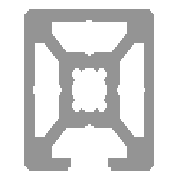
# Autodesk Inventor part: 3 842 993 421-25mm
Saved by Autodesk Inventor 2011 SP1 (Build 150282100, 282)
## iProperties
Created: 2011-02-10
Part Number: 3 842 993 421-25mm
Document SubType Name: Modeling
Designer: S. Wile
Density: 2.71 g/cm^3
Categories: <MemberInstance><Categories><Category DisplayName="Structural Shapes" InternalName="089c4875-fa83-4c05-b084-43b9cc11f5ed" Mnemonic="GRDR"><CategoryParameter DisplayName="Custom Base Point" InternalName="4f1d1b73-316d-484b-a3df-9cbabb16eb77" Mnemonic="shpBasePoint"/><CategoryParameter DisplayName="FG Authored" InternalName="9c666724-f362-4ea7-ac62-f6a007de5c69" Mnemonic="shpFGAuto"/><CategoryParameter DisplayName="Legacy Member ID" InternalName="340afe4f-75d7-48d3-ab7d-943f3c3da468" Mnemonic="LegacyMemberID"/><CategoryParameter DisplayName="Base Length" InternalName="42e34263-8f20-4d0e-ad48-bf1385b87c24" Mnemonic="shplen"/><CategoryParameter DisplayName="Distance of the Center of Gravity X-X" InternalName="26c9bdb8-9c79-4b4f-a92e-8e197583c9c4" Mnemonic="grcendistX"/><CategoryParameter DisplayName="Distance of the Center of Gravity Y-Y" InternalName="bcc4fb17-7af4-436a-8f8c-d0aa3b0248c5" Mnemonic="grcendistY"/><CategoryParameter DisplayName="Torsional Rigidity Modulus" InternalName="26c1ec35-5026-4c63-ad0a-751cf684a536" Mnemonic="torrigmod"/><CategoryParameter DisplayName="Torsional Section Modulus" InternalName="7c55a8dc-8844-49f9-a867-cc677b30ec9a" Mnemonic="torsecmod"/><CategoryParameter DisplayName="Coefficient of Shear Displacement" InternalName="de4c90c6-aaa8-468f-a335-6737b311b5d3" Mnemonic="shdispc"/><CategoryParameter DisplayName="Section Area" InternalName="1ff91680-64b0-4202-b9a3-7fd3f94bba3b" Mnemonic="secarea"/><CategoryParameter DisplayName="Moment of Inertia (x)" InternalName="4cd780bc-73d7-43ac-917a-579e5cbd684d" Mnemonic="inermomx"/><CategoryParameter DisplayName="Moment of Inertia (y)" InternalName="4b9f58ea-bced-460e-81ea-3d29ca5a49e3" Mnemonic="inermomy"/><CategoryParameter DisplayName="Section Module (x)" InternalName="72cfad18-cf51-4ed4-aaa7-c6b224f8419f" Mnemonic="secmodx"/><CategoryParameter DisplayName="Section Module (y)" InternalName="59eaa5e9-d227-48dc-b6c1-6920f96e0f95" Mnemonic="secmody"/><CategoryParameter DisplayName="Radius of Gyration (x)" InternalName="25778675-03e9-40c1-b6a8-4a9ed693320d" Mnemonic="gyrradx"/><CategoryParameter DisplayName="Radius of Gyration (y)" InternalName="bfa18ebe-1636-4dbe-8d42-b263e0b73184" Mnemonic="gyrrady"/><CategoryParameter DisplayName="Shape Thickness" InternalName="d109cf76-8eb4-42fc-9800-4409734adc67" Mnemonic="shpthick"/><CategoryParameter DisplayName="Second Shape Thickness" InternalName="9251a8e1-85fd-4e47-af99-afdb762317d9" Mnemonic="shpthick2"/><CategoryParameter DisplayName="Shape Width" InternalName="7c717d54-a18f-4666-b4d4-573cce22c62c" Mnemonic="shpwdth"/><CategoryParameter DisplayName="Shape Height" InternalName="50274e7d-5ac0-4796-92cb-c59e54983c67" Mnemonic="shpheig"/><CategoryParameter DisplayName="Mass per Length Unit" InternalName="0bb95a10-148f-4027-a459-38d7b056702a" Mnemonic="shpmass"/><CategoryParameter DisplayName="Section Designation" InternalName="5a64d034-428d-49c8-ba32-7619764de20f" Mnemonic="shpdes"/><Category DisplayName="Other" InternalName="f02205ff-2390-476f-921c-0b3185f88e84" Mnemonic="OTHSHP"><CategoryParameter DisplayName="Moment of Inertia (x)" InternalName="ec6737bc-264f-43ed-b0bd-f6d410c2718d" Mnemonic="inermomx"/><CategoryParameter DisplayName="Moment of Inertia (y)" InternalName="044c654e-f649-48ac-84cc-650a29ae31ca" Mnemonic="inermomy"/><CategoryParameter DisplayName="Section Module (x)" InternalName="cac70804-9d39-43bb-be17-56ea1f39a6c2" Mnemonic="secmodx"/><CategoryParameter DisplayName="Section Module (y)" InternalName="88b8bff9-a616-4028-93d5-ed4f79680d13" Mnemonic="secmody"/><CategoryParameter DisplayName="Section Area" InternalName="c46ecdf8-b6eb-4db9-8b25-30258930c1e3" Mnemonic="secarea"/><CategoryParameter DisplayName="Radius of Gyration (x)" InternalName="ee72c61e-565e-4fd6-b448-66e1e1abcb7e" Mnemonic="gyrradx"/><CategoryParameter DisplayName="Radius of Gyration (y)" InternalName="743e1dfe-1bba-408b-b985-cf752b207386" Mnemonic="gyrrady"/><CategoryParameter DisplayName="Shape Thickness" InternalName="12b1a788-9233-48fd-a933-2df8ff42b15f" Mnemonic="shpthick"/><CategoryParameter DisplayName="Mass per Length Unit" InternalName="2fd289d6-9394-4d2d-97e6-6659d7d4551d" Mnemonic="shpmass"/></Category></Category></Categories><FamilyTemplate Id="20x20-1S"><FamilyTemplateParameters><FamilyTemplateParameter ObjectType="kUserParameterObject" ValueType="xs:double" Id="1" ObjectReferenceKey="Length"/><FamilyTemplateParameter ObjectType="kPropertyObject" ValueType="xs:string" Id="4" ObjectReferenceKey="{32853F0F-3444-11d1-9E93-0060B03C1CA6}" SubObjectId="52"/><FamilyTemplateParameter ObjectType="kPartComponentDefinitionObject" ValueType="xs:string" Id="5" SubObjectId="Material"/><FamilyTemplateParameter ObjectType="kPropertyObject" ValueType="xs:string" Id="6" ObjectReferenceKey="{32853F0F-3444-11d1-9E93-0060B03C1CA6}" SubObjectId="5"/><FamilyTemplateParameter ObjectType="kPropertyObject" ValueType="xs:string" Id="7" ObjectReferenceKey="{32853F0F-3444-11D1-9E93-0060B03C1CA6}" SubObjectId="55"/><FamilyTemplateParameter ObjectType="kiPartTableColumnObject" ValueType="xs:string" Id="16" ObjectReferenceKey="FILENAME"/><FamilyTemplateParameter ObjectType="kiPartTableColumnObject" ValueType="xs:string" Id="17" ObjectReferenceKey="MEMBER_REVISION"/></FamilyTemplateParameters></FamilyTemplate><CategoryParameterMap><ParamToTemplateMap><ParamToTemplate CategoryParameter="//CategoryParameter[@InternalName='2675968c-4ce5-49e0-a4f5-552d29089031']" TemplateParameter="4"/><ParamToTemplate CategoryParameter="//CategoryParameter[@InternalName='8b46a4cc-9585-4fed-90c3-899f57e09a73']" TemplateParameter="16"/><ParamToTemplate CategoryParameter="//CategoryParameter[@InternalName='42e34263-8f20-4d0e-ad48-bf1385b87c24']" TemplateParameter="1"/><ParamToTemplate CategoryParameter="//CategoryParameter[@InternalName='818a152a-d3c3-49ca-80ee-df7d91421b8e']" TemplateParameter="5"/><ParamToTemplate CategoryParameter="//CategoryParameter[@InternalName='a65d44b9-392f-4f4f-857b-e4b3d54996fe']" TemplateParameter="17"/><ParamToTemplate CategoryParameter="//CategoryParameter[@InternalName='016b6077-bfbe-49bd-92c9-d8d59c39c941']" TemplateParameter="6"/><ParamToTemplate CategoryParameter="//CategoryParameter[@InternalName='9c666724-f362-4ea7-ac62-f6a007de5c69']" ConstantValue="1"/></ParamToTemplateMap></CategoryParameterMap></MemberInstance>
Stock Number: 3 842 993 421
Description: PROFILE 20x20 1S, -/-
Material: Aluminum-6061
Mass: 13.0174 g
Surface Area: 55.674 cm^2
Volume: 4.80347 cm^3
Author: S. Wile
Autodesk Inventor part; units mm, degrees
ref_plane "YZ Plane" through (0, 0, 0) normal (1, 0, 0) x (0, 1, 0)
ref_plane "XZ Plane" through (0, 0, 0) normal (0, 1, 0) x (-1, 0, 0)
ref_plane "XY Plane" through (0, 0, 0) normal (0, 0, 1) x (1, 0, 0)
sketch "20x20-1S" plane through (0, 0, 0) normal (0, 0, 1) x (1, 0, 0)
  arc A0 (162.0009, 79.9596) -> (163.0616, 81.0203) centre (160.1138, 82.9073) ccw
  line L0 (163.0616, 81.0203) -> (162.5495, 81.6306)
  arc A1 (162.5495, 81.6306) -> (162.5495, 84.184) centre (160.1138, 82.9073) ccw
  line L1 (162.5495, 84.184) -> (163.0616, 84.7943)
  arc A2 (163.0616, 84.7943) -> (162.0009, 85.855) centre (160.1138, 82.9073) ccw
  line L2 (162.0009, 85.855) -> (161.3907, 85.3429)
  arc A3 (161.3907, 85.3429) -> (158.8369, 85.3429) centre (160.1138, 82.9073) ccw
  line L3 (158.8369, 85.3429) -> (158.2267, 85.855)
  arc A4 (158.2267, 85.855) -> (157.166, 84.7943) centre (160.1138, 82.9073) ccw
  line L4 (157.166, 84.7943) -> (157.6781, 84.184)
  arc A5 (157.6781, 84.184) -> (157.6781, 81.6306) centre (160.1138, 82.9073) ccw
  line L5 (157.6781, 81.6306) -> (157.166, 81.0203)
  arc A6 (157.166, 81.0203) -> (158.2267, 79.9596) centre (160.1138, 82.9073) ccw
  line L6 (158.2267, 79.9596) -> (158.8369, 80.4717)
  arc A7 (158.8369, 80.4717) -> (161.3907, 80.4717) centre (160.1138, 82.9073) ccw
  line L7 (161.3907, 80.4717) -> (162.0009, 79.9596)
  line L8 (164.6138, 81.9877) -> (164.6138, 79.5508)
  line L9 (164.6724, 79.4094) -> (167.1159, 76.9659)
  line L10 (167.2573, 76.9073) -> (168.4138, 76.9073)
  line L11 (168.6138, 77.1073) -> (168.6138, 82.3341)
  line L12 (168.6406, 82.4341) -> (168.8561, 82.8073)
  line L13 (168.8561, 83.0073) -> (168.6406, 83.3805)
  line L14 (168.6138, 83.4805) -> (168.6138, 88.7073)
  line L15 (168.4138, 88.9073) -> (167.2573, 88.9073)
  line L16 (167.1159, 88.8487) -> (164.6724, 86.4052)
  line L17 (164.6138, 86.2638) -> (164.6138, 83.8269)
  line L18 (164.587, 83.7269) -> (164.1715, 83.0073)
  line L19 (164.1715, 82.8073) -> (164.587, 82.0877)
  line L20 (161.0334, 87.4073) -> (163.4703, 87.4073)
  line L21 (166.1138, 90.0508) -> (166.1138, 91.2073)
  line L22 (165.9138, 91.4073) -> (160.687, 91.4073)
  line L23 (160.587, 91.4341) -> (160.2138, 91.6495)
  line L24 (160.0138, 91.6495) -> (159.6406, 91.4341)
  line L25 (159.5406, 91.4073) -> (154.3138, 91.4073)
  line L26 (154.1138, 91.2073) -> (154.1138, 90.0508)
  line L27 (154.1724, 89.9094) -> (156.6159, 87.4659)
  line L28 (156.7573, 87.4073) -> (159.1942, 87.4073)
  line L29 (159.2942, 87.3805) -> (160.0138, 86.965)
  line L30 (160.2138, 86.965) -> (160.9334, 87.3805)
  line L31 (155.6138, 83.8269) -> (155.6138, 86.2638)
  line L32 (155.5552, 86.4052) -> (153.1117, 88.8487)
  line L33 (152.9703, 88.9073) -> (151.8138, 88.9073)
  line L34 (151.6138, 88.7073) -> (151.6138, 83.4805)
  line L35 (151.587, 83.3805) -> (151.3715, 83.0073)
  line L36 (151.3715, 82.8073) -> (151.587, 82.4341)
  line L37 (151.6138, 82.3341) -> (151.6138, 77.1073)
  line L38 (151.8138, 76.9073) -> (152.9703, 76.9073)
  line L39 (153.1117, 76.9659) -> (155.5552, 79.4094)
  line L40 (155.6138, 79.5508) -> (155.6138, 81.9877)
  line L41 (155.6406, 82.0877) -> (156.0561, 82.8073)
  line L42 (156.0561, 83.0073) -> (155.6406, 83.7269)
  line L43 (163.6117, 87.4659) -> (166.0552, 89.9094)
  line L44 (150.1138, 91.4073) -> (150.1138, 74.4073)
  arc A8 (150.1138, 74.4073) -> (151.6138, 72.9073) centre (151.6138, 74.4073) ccw
  line L45 (151.6138, 72.9073) -> (156.4138, 72.9073)
  line L46 (156.6138, 73.1073) -> (156.6138, 73.2073)
  line L47 (156.8138, 73.4073) -> (156.9138, 73.4073)
  line L48 (157.1138, 73.6073) -> (157.1138, 74.2073)
  line L49 (156.9138, 74.4073) -> (154.3138, 74.4073)
  line L50 (154.1138, 74.6073) -> (154.1138, 75.7638)
  line L51 (154.1724, 75.9052) -> (156.6159, 78.3487)
  line L52 (156.7573, 78.4073) -> (159.1942, 78.4073)
  line L53 (159.2942, 78.4341) -> (160.0138, 78.8495)
  line L54 (160.2138, 78.8495) -> (160.9334, 78.4341)
  line L55 (161.0334, 78.4073) -> (163.4703, 78.4073)
  line L56 (163.6117, 78.3487) -> (166.0552, 75.9052)
  line L57 (166.1138, 75.7638) -> (166.1138, 74.6073)
  line L58 (165.9138, 74.4073) -> (163.3138, 74.4073)
  line L59 (163.1138, 74.2073) -> (163.1138, 73.6073)
  line L60 (163.3138, 73.4073) -> (163.4138, 73.4073)
  line L61 (163.6138, 73.2073) -> (163.6138, 73.1073)
  line L62 (163.8138, 72.9073) -> (168.6138, 72.9073)
  arc A9 (168.6138, 72.9073) -> (170.1138, 74.4073) centre (168.6138, 74.4073) ccw
  line L63 (170.1138, 74.4073) -> (170.1138, 91.4073)
  arc A10 (170.1138, 91.4073) -> (168.6138, 92.9073) centre (168.6138, 91.4073) ccw
  line L64 (168.6138, 92.9073) -> (151.6138, 92.9073)
  arc A11 (151.6138, 92.9073) -> (150.1138, 91.4073) centre (151.6138, 91.4073) ccw
  arc A12 (151.8138, 88.9073) -> (151.6138, 88.7073) centre (151.8138, 88.7073) ccw
  arc A13 (153.1117, 88.8487) -> (152.9703, 88.9073) centre (152.9703, 88.7073) ccw
  arc A14 (155.6138, 86.2638) -> (155.5552, 86.4052) centre (155.4138, 86.2638) ccw
  arc A15 (155.6138, 83.8269) -> (155.6406, 83.7269) centre (155.8138, 83.8269) ccw
  arc A16 (156.0561, 82.8073) -> (156.0561, 83.0073) centre (155.8829, 82.9073) ccw
  arc A17 (155.6406, 82.0877) -> (155.6138, 81.9877) centre (155.8138, 81.9877) ccw
  arc A18 (151.3715, 83.0073) -> (151.3715, 82.8073) centre (151.5447, 82.9073) ccw
  arc A19 (151.587, 83.3805) -> (151.6138, 83.4805) centre (151.4138, 83.4805) ccw
  arc A20 (151.6138, 82.3341) -> (151.587, 82.4341) centre (151.4138, 82.3341) ccw
  arc A21 (152.9703, 76.9073) -> (153.1117, 76.9659) centre (152.9703, 77.1073) ccw
  arc A22 (151.6138, 77.1073) -> (151.8138, 76.9073) centre (151.8138, 77.1073) ccw
  arc A23 (155.5552, 79.4094) -> (155.6138, 79.5508) centre (155.4138, 79.5508) ccw
  arc A24 (154.1138, 74.6073) -> (154.3138, 74.4073) centre (154.3138, 74.6073) ccw
  arc A25 (154.1724, 75.9052) -> (154.1138, 75.7638) centre (154.3138, 75.7638) ccw
  arc A26 (156.7573, 78.4073) -> (156.6159, 78.3487) centre (156.7573, 78.2073) ccw
  arc A27 (159.1942, 78.4073) -> (159.2942, 78.4341) centre (159.1942, 78.6073) ccw
  arc A28 (160.2138, 78.8495) -> (160.0138, 78.8495) centre (160.1138, 78.6763) ccw
  arc A29 (160.9334, 78.4341) -> (161.0334, 78.4073) centre (161.0334, 78.6073) ccw
  arc A30 (163.6117, 78.3487) -> (163.4703, 78.4073) centre (163.4703, 78.2073) ccw
  arc A31 (157.1138, 74.2073) -> (156.9138, 74.4073) centre (156.9138, 74.2073) ccw
  arc A32 (156.9138, 73.4073) -> (157.1138, 73.6073) centre (156.9138, 73.6073) ccw
  arc A33 (156.8138, 73.4073) -> (156.6138, 73.2073) centre (156.8138, 73.2073) ccw
  arc A34 (156.4138, 72.9073) -> (156.6138, 73.1073) centre (156.4138, 73.1073) ccw
  arc A35 (163.6138, 73.1073) -> (163.8138, 72.9073) centre (163.8138, 73.1073) ccw
  arc A36 (163.6138, 73.2073) -> (163.4138, 73.4073) centre (163.4138, 73.2073) ccw
  arc A37 (163.1138, 73.6073) -> (163.3138, 73.4073) centre (163.3138, 73.6073) ccw
  arc A38 (163.3138, 74.4073) -> (163.1138, 74.2073) centre (163.3138, 74.2073) ccw
  arc A39 (165.9138, 74.4073) -> (166.1138, 74.6073) centre (165.9138, 74.6073) ccw
  arc A40 (166.1138, 75.7638) -> (166.0552, 75.9052) centre (165.9138, 75.7638) ccw
  arc A41 (167.1159, 76.9659) -> (167.2573, 76.9073) centre (167.2573, 77.1073) ccw
  arc A42 (168.4138, 76.9073) -> (168.6138, 77.1073) centre (168.4138, 77.1073) ccw
  arc A43 (164.6138, 79.5508) -> (164.6724, 79.4094) centre (164.8138, 79.5508) ccw
  arc A44 (164.6138, 81.9877) -> (164.587, 82.0877) centre (164.4138, 81.9877) ccw
  arc A45 (164.1715, 83.0073) -> (164.1715, 82.8073) centre (164.3447, 82.9073) ccw
  arc A46 (164.587, 83.7269) -> (164.6138, 83.8269) centre (164.4138, 83.8269) ccw
  arc A47 (168.8561, 82.8073) -> (168.8561, 83.0073) centre (168.6829, 82.9073) ccw
  arc A48 (168.6406, 82.4341) -> (168.6138, 82.3341) centre (168.8138, 82.3341) ccw
  arc A49 (168.6138, 83.4805) -> (168.6406, 83.3805) centre (168.8138, 83.4805) ccw
  arc A50 (164.6724, 86.4052) -> (164.6138, 86.2638) centre (164.8138, 86.2638) ccw
  arc A51 (167.2573, 88.9073) -> (167.1159, 88.8487) centre (167.2573, 88.7073) ccw
  arc A52 (168.6138, 88.7073) -> (168.4138, 88.9073) centre (168.4138, 88.7073) ccw
  arc A53 (166.0552, 89.9094) -> (166.1138, 90.0508) centre (165.9138, 90.0508) ccw
  arc A54 (163.4703, 87.4073) -> (163.6117, 87.4659) centre (163.4703, 87.6073) ccw
  arc A55 (160.0138, 86.965) -> (160.2138, 86.965) centre (160.1138, 87.1382) ccw
  arc A56 (161.0334, 87.4073) -> (160.9334, 87.3805) centre (161.0334, 87.2073) ccw
  arc A57 (159.2942, 87.3805) -> (159.1942, 87.4073) centre (159.1942, 87.2073) ccw
  arc A58 (159.5406, 91.4073) -> (159.6406, 91.4341) centre (159.5406, 91.6073) ccw
  arc A59 (160.2138, 91.6495) -> (160.0138, 91.6495) centre (160.1138, 91.4763) ccw
  arc A60 (160.587, 91.4341) -> (160.687, 91.4073) centre (160.687, 91.6073) ccw
  arc A61 (166.1138, 91.2073) -> (165.9138, 91.4073) centre (165.9138, 91.2073) ccw
  arc A62 (156.6159, 87.4659) -> (156.7573, 87.4073) centre (156.7573, 87.6073) ccw
  arc A63 (154.1138, 90.0508) -> (154.1724, 89.9094) centre (154.3138, 90.0508) ccw
  arc A64 (154.3138, 91.4073) -> (154.1138, 91.2073) centre (154.3138, 91.2073) ccw
  dimension "d0" = 0.2
  dimension "d1" = 0.2
  dimension "d2" = 0.2
  measures "d0" radius of A12
  measures "d1" radius of A27
  measures "d2" radius of A50
sketch "Sketch1" plane through (0, 0, 0) normal (0, 0, 1) x (1, 0, 0)
  arc A0 (1.8871, -2.9477) -> (2.9478, -1.887) centre (0, 0) ccw
  line L0 (2.9478, -1.887) -> (2.4357, -1.2767)
  arc A1 (2.4357, -1.2767) -> (2.4357, 1.2767) centre (0, 0) ccw
  line L1 (2.4357, 1.2767) -> (2.9478, 1.887)
  arc A2 (2.9478, 1.887) -> (1.8871, 2.9477) centre (0, 0) ccw
  line L2 (1.8871, 2.9477) -> (1.2769, 2.4356)
  arc A3 (1.2769, 2.4356) -> (-1.2769, 2.4356) centre (0, 0) ccw
  line L3 (-1.2769, 2.4356) -> (-1.8871, 2.9477)
  arc A4 (-1.8871, 2.9477) -> (-2.9478, 1.887) centre (0, 0) ccw
  line L4 (-2.9478, 1.887) -> (-2.4357, 1.2767)
  arc A5 (-2.4357, 1.2767) -> (-2.4357, -1.2767) centre (0, 0) ccw
  line L5 (-2.4357, -1.2767) -> (-2.9478, -1.887)
  arc A6 (-2.9478, -1.887) -> (-1.8871, -2.9477) centre (0, 0) ccw
  line L6 (-1.8871, -2.9477) -> (-1.2769, -2.4356)
  arc A7 (-1.2769, -2.4356) -> (1.2769, -2.4356) centre (0, 0) ccw
  line L7 (1.2769, -2.4356) -> (1.8871, -2.9477)
  line L8 (4.5, -0.9196) -> (4.5, -3.3565)
  line L9 (4.5586, -3.4979) -> (7.0021, -5.9414)
  line L10 (7.1435, -6) -> (8.3, -6)
  line L11 (8.5, -5.8) -> (8.5, -0.5732)
  line L12 (8.5268, -0.4732) -> (8.7423, -0.1)
  line L13 (8.7423, 0.1) -> (8.5268, 0.4732)
  line L14 (8.5, 0.5732) -> (8.5, 5.8)
  line L15 (8.3, 6) -> (7.1435, 6)
  line L16 (7.0021, 5.9414) -> (4.5586, 3.4979)
  line L17 (4.5, 3.3565) -> (4.5, 0.9196)
  line L18 (4.4732, 0.8196) -> (4.0577, 0.1)
  line L19 (4.0577, -0.1) -> (4.4732, -0.8196)
  line L20 (0.9196, 4.5) -> (3.3565, 4.5)
  line L21 (6, 7.1435) -> (6, 8.3)
  line L22 (5.8, 8.5) -> (0.5732, 8.5)
  line L23 (0.4732, 8.5268) -> (0.1, 8.7423)
  line L24 (-0.1, 8.7423) -> (-0.4732, 8.5268)
  line L25 (-0.5732, 8.5) -> (-5.8, 8.5)
  line L26 (-6, 8.3) -> (-6, 7.1435)
  line L27 (-5.9414, 7.0021) -> (-3.4979, 4.5586)
  line L28 (-3.3565, 4.5) -> (-0.9196, 4.5)
  line L29 (-0.8196, 4.4732) -> (-0.1, 4.0577)
  line L30 (0.1, 4.0577) -> (0.8196, 4.4732)
  line L31 (-4.5, 0.9196) -> (-4.5, 3.3565)
  line L32 (-4.5586, 3.4979) -> (-7.0021, 5.9414)
  line L33 (-7.1435, 6) -> (-8.3, 6)
  line L34 (-8.5, 5.8) -> (-8.5, 0.5732)
  line L35 (-8.5268, 0.4732) -> (-8.7423, 0.1)
  line L36 (-8.7423, -0.1) -> (-8.5268, -0.4732)
  line L37 (-8.5, -0.5732) -> (-8.5, -5.8)
  line L38 (-8.3, -6) -> (-7.1435, -6)
  line L39 (-7.0021, -5.9414) -> (-4.5586, -3.4979)
  line L40 (-4.5, -3.3565) -> (-4.5, -0.9196)
  line L41 (-4.4732, -0.8196) -> (-4.0577, -0.1)
  line L42 (-4.0577, 0.1) -> (-4.4732, 0.8196)
  line L43 (3.4979, 4.5586) -> (5.9414, 7.0021)
  line L44 (-10, 8.5) -> (-10, -8.5)
  arc A8 (-10, -8.5) -> (-8.5, -10) centre (-8.5, -8.5) ccw
  line L45 (-8.5, -10) -> (-3.7, -10)
  line L46 (-3.5, -9.8) -> (-3.5, -9.7)
  line L47 (-3.3, -9.5) -> (-3.2, -9.5)
  line L48 (-3, -9.3) -> (-3, -8.7)
  line L49 (-3.2, -8.5) -> (-5.8, -8.5)
  line L50 (-6, -8.3) -> (-6, -7.1435)
  line L51 (-5.9414, -7.0021) -> (-3.4979, -4.5586)
  line L52 (-3.3565, -4.5) -> (-0.9196, -4.5)
  line L53 (-0.8196, -4.4732) -> (-0.1, -4.0577)
  line L54 (0.1, -4.0577) -> (0.8196, -4.4732)
  line L55 (0.9196, -4.5) -> (3.3565, -4.5)
  line L56 (3.4979, -4.5586) -> (5.9414, -7.0021)
  line L57 (6, -7.1435) -> (6, -8.3)
  line L58 (5.8, -8.5) -> (3.2, -8.5)
  line L59 (3, -8.7) -> (3, -9.3)
  line L60 (3.2, -9.5) -> (3.3, -9.5)
  line L61 (3.5, -9.7) -> (3.5, -9.8)
  line L62 (3.7, -10) -> (8.5, -10)
  arc A9 (8.5, -10) -> (10, -8.5) centre (8.5, -8.5) ccw
  line L63 (10, -8.5) -> (10, 8.5)
  arc A10 (10, 8.5) -> (8.5, 10) centre (8.5, 8.5) ccw
  line L64 (8.5, 10) -> (-8.5, 10)
  arc A11 (-8.5, 10) -> (-10, 8.5) centre (-8.5, 8.5) ccw
  arc A12 (-8.3, 6) -> (-8.5, 5.8) centre (-8.3, 5.8) ccw
  arc A13 (-7.0021, 5.9414) -> (-7.1435, 6) centre (-7.1435, 5.8) ccw
  arc A14 (-4.5, 3.3565) -> (-4.5586, 3.4979) centre (-4.7, 3.3565) ccw
  arc A15 (-4.5, 0.9196) -> (-4.4732, 0.8196) centre (-4.3, 0.9196) ccw
  arc A16 (-4.0577, -0.1) -> (-4.0577, 0.1) centre (-4.2309, 0) ccw
  arc A17 (-4.4732, -0.8196) -> (-4.5, -0.9196) centre (-4.3, -0.9196) ccw
  arc A18 (-8.7423, 0.1) -> (-8.7423, -0.1) centre (-8.5691, 0) ccw
  arc A19 (-8.5268, 0.4732) -> (-8.5, 0.5732) centre (-8.7, 0.5732) ccw
  arc A20 (-8.5, -0.5732) -> (-8.5268, -0.4732) centre (-8.7, -0.5732) ccw
  arc A21 (-7.1435, -6) -> (-7.0021, -5.9414) centre (-7.1435, -5.8) ccw
  arc A22 (-8.5, -5.8) -> (-8.3, -6) centre (-8.3, -5.8) ccw
  arc A23 (-4.5586, -3.4979) -> (-4.5, -3.3565) centre (-4.7, -3.3565) ccw
  arc A24 (-6, -8.3) -> (-5.8, -8.5) centre (-5.8, -8.3) ccw
  arc A25 (-5.9414, -7.0021) -> (-6, -7.1435) centre (-5.8, -7.1435) ccw
  arc A26 (-3.3565, -4.5) -> (-3.4979, -4.5586) centre (-3.3565, -4.7) ccw
  arc A27 (-0.9196, -4.5) -> (-0.8196, -4.4732) centre (-0.9196, -4.3) ccw
  arc A28 (0.1, -4.0577) -> (-0.1, -4.0577) centre (0, -4.2309) ccw
  arc A29 (0.8196, -4.4732) -> (0.9196, -4.5) centre (0.9196, -4.3) ccw
  arc A30 (3.4979, -4.5586) -> (3.3565, -4.5) centre (3.3565, -4.7) ccw
  arc A31 (-3, -8.7) -> (-3.2, -8.5) centre (-3.2, -8.7) ccw
  arc A32 (-3.2, -9.5) -> (-3, -9.3) centre (-3.2, -9.3) ccw
  arc A33 (-3.3, -9.5) -> (-3.5, -9.7) centre (-3.3, -9.7) ccw
  arc A34 (-3.7, -10) -> (-3.5, -9.8) centre (-3.7, -9.8) ccw
  arc A35 (3.5, -9.8) -> (3.7, -10) centre (3.7, -9.8) ccw
  arc A36 (3.5, -9.7) -> (3.3, -9.5) centre (3.3, -9.7) ccw
  arc A37 (3, -9.3) -> (3.2, -9.5) centre (3.2, -9.3) ccw
  arc A38 (3.2, -8.5) -> (3, -8.7) centre (3.2, -8.7) ccw
  arc A39 (5.8, -8.5) -> (6, -8.3) centre (5.8, -8.3) ccw
  arc A40 (6, -7.1435) -> (5.9414, -7.0021) centre (5.8, -7.1435) ccw
  arc A41 (7.0021, -5.9414) -> (7.1435, -6) centre (7.1435, -5.8) ccw
  arc A42 (8.3, -6) -> (8.5, -5.8) centre (8.3, -5.8) ccw
  arc A43 (4.5, -3.3565) -> (4.5586, -3.4979) centre (4.7, -3.3565) ccw
  arc A44 (4.5, -0.9196) -> (4.4732, -0.8196) centre (4.3, -0.9196) ccw
  arc A45 (4.0577, 0.1) -> (4.0577, -0.1) centre (4.2309, 0) ccw
  arc A46 (4.4732, 0.8196) -> (4.5, 0.9196) centre (4.3, 0.9196) ccw
  arc A47 (8.7423, -0.1) -> (8.7423, 0.1) centre (8.5691, 0) ccw
  arc A48 (8.5268, -0.4732) -> (8.5, -0.5732) centre (8.7, -0.5732) ccw
  arc A49 (8.5, 0.5732) -> (8.5268, 0.4732) centre (8.7, 0.5732) ccw
  arc A50 (4.5586, 3.4979) -> (4.5, 3.3565) centre (4.7, 3.3565) ccw
  arc A51 (7.1435, 6) -> (7.0021, 5.9414) centre (7.1435, 5.8) ccw
  arc A52 (8.5, 5.8) -> (8.3, 6) centre (8.3, 5.8) ccw
  arc A53 (5.9414, 7.0021) -> (6, 7.1435) centre (5.8, 7.1435) ccw
  arc A54 (3.3565, 4.5) -> (3.4979, 4.5586) centre (3.3565, 4.7) ccw
  arc A55 (-0.1, 4.0577) -> (0.1, 4.0577) centre (0, 4.2309) ccw
  arc A56 (0.9196, 4.5) -> (0.8196, 4.4732) centre (0.9196, 4.3) ccw
  arc A57 (-0.8196, 4.4732) -> (-0.9196, 4.5) centre (-0.9196, 4.3) ccw
  arc A58 (-0.5732, 8.5) -> (-0.4732, 8.5268) centre (-0.5732, 8.7) ccw
  arc A59 (0.1, 8.7423) -> (-0.1, 8.7423) centre (0, 8.5691) ccw
  arc A60 (0.4732, 8.5268) -> (0.5732, 8.5) centre (0.5732, 8.7) ccw
  arc A61 (6, 8.3) -> (5.8, 8.5) centre (5.8, 8.3) ccw
  arc A62 (-3.4979, 4.5586) -> (-3.3565, 4.5) centre (-3.3565, 4.7) ccw
  arc A63 (-6, 7.1435) -> (-5.9414, 7.0021) centre (-5.8, 7.1435) ccw
  arc A64 (-5.8, 8.5) -> (-6, 8.3) centre (-5.8, 8.3) ccw
  constraints: 1 other
extrude "Extrusion3" add sketch "Sketch1" along normal blind 30
body "Solid2"
